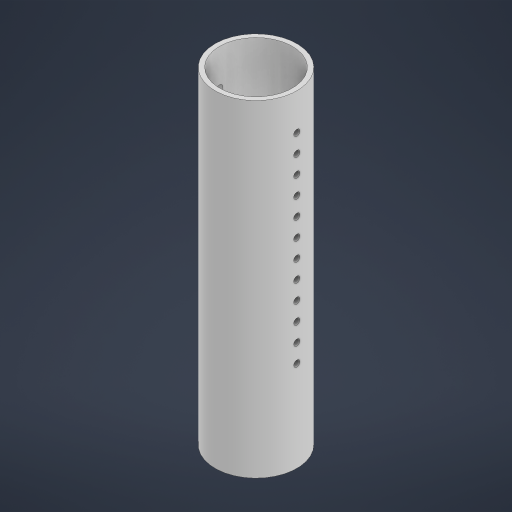
# Autodesk Inventor part: Air Chamber
Saved by Autodesk Inventor 2024.1 (Build 281209000, 209)
## iProperties
Created: 2024-11-18
Part Number: Air Chamber
Material: Generic
Document SubType Name: Modeling
Designer: Designer
Density: 1 g/cm^3
Appearance: Default
Author: Designer
Autodesk Inventor part; units mm, degrees
ref_plane "XZ Plane" through (0, 0, 0) normal (0, 1, 0) x (-1, 0, 0)
ref_plane "XY Plane" through (0, 0, 0) normal (0, 0, 1) x (1, 0, 0)
sketch "Sketch1" plane through (0, 0, 0) normal (0, 1, 0) x (-1, 0, 0)
  circle A0 centre (0, 0) radius 50.8
  circle A1 centre (0, 0) radius 57.15
  dimension "d1" = 101.6
  dimension "d2" = 114.3
  constraints: 2 centre point, 2 coincident
  measures "d1" diameter of A0
  measures "d2" diameter of A1
extrude "Extrusion1" add sketch "Sketch1" along normal blind 457.2
ref_plane "Work Plane1" through (-57.15, 0, 0) normal (1, 0, 0) x (0, 1, 0)
sketch "Sketch2" plane through (-57.15, 0, 0) normal (1, 0, 0) x (0, 1, 0)
  line L0 (0, 0) -> (457.2, 0) construction
  line L1 (457.2, -57.15) -> (457.2, 57.15) construction
  circle A0 centre (406.4, 0) radius 4.25
  circle A1 centre (381, 0) radius 4.25
  circle A2 centre (330.2, 0) radius 4.25
  circle A3 centre (355.6, 0) radius 4.25
  circle A4 centre (304.8, 0) radius 4.25
  circle A5 centre (279.4, 0) radius 4.25
  circle A6 centre (177.8, 0) radius 4.25
  circle A7 centre (254, 0) radius 4.25
  circle A8 centre (228.6, 0) radius 4.25
  circle A9 centre (203.2, 0) radius 4.25
  circle A10 centre (152.4, 0) radius 4.25
  circle A11 centre (127, 0) radius 4.25
  point P0 (228.6, 0)
  dimension "d6" = 50.8
  dimension "d7" = 25.4
  dimension "d8" = 25.4
  dimension "d9" = 25.4
  dimension "d10" = 25.4
  dimension "d11" = 25.4
  dimension "d12" = 25.4
  dimension "d13" = 25.4
  dimension "d14" = 25.4
  dimension "d15" = 25.4
  dimension "d16" = 25.4
  dimension "d17" = 25.4
  dimension "d18" = 8.5
  constraints: 12 centre point, 11 equal radius, 1 midpoint, 16 other
  measures "d6" distance from line of L1 A0.centre
  measures "d7" distance of A0.centre A1.centre
  measures "d8" distance of A3.centre A1.centre
  measures "d9" distance of A2.centre A3.centre
  measures "d10" distance of A2.centre A4.centre
  measures "d11" distance of A4.centre A5.centre
  measures "d12" distance of A5.centre A7.centre
  measures "d13" distance of A7.centre A8.centre
  measures "d14" distance of point (228.6, 0) A9.centre
  measures "d15" distance of A9.centre A6.centre
  measures "d16" distance of A6.centre A10.centre
  measures "d17" distance of A10.centre A11.centre
  measures "d18" diameter of A0
extrude "Extrusion2" cut sketch "Sketch2" along normal blind 457.2
body "Solid1"
